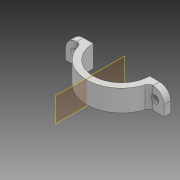
# Autodesk Inventor part: bottom_fitting
Saved by Autodesk Inventor 2017 (Build 210142000, 142)
## iProperties
Created: 2017-06-10
Part Number: bottom_fitting
Material: Generic
Document SubType Name: Modeling
Designer: ari
Density: 1 g/cm^3
Appearance: Default
Author: ari
Autodesk Inventor part; units mm, degrees
ref_plane "YZ Plane" through (0, 0, 0) normal (1, 0, 0) x (0, 1, 0)
ref_plane "XZ Plane" through (0, 0, 0) normal (0, 1, 0) x (-1, 0, 0)
ref_plane "XY Plane" through (0, 0, 0) normal (0, 0, 1) x (1, 0, 0)
sketch "Sketch1" plane through (0, 0, 0) normal (0, 0, 1) x (1, 0, 0)
  line L0 (12.7, 0) -> (22.2, 0)
  line L1 (22.2, 0) -> (22.2, -3)
  line L2 (22.2, -3) -> (12.7, -3)
  line L3 (12.7, -3) -> (12.7, 0)
  circle A0 centre (0, 0) radius 12.7
  circle A1 centre (0, 0) radius 15.7
  line L4 (-15.7, 0) -> (-12.7, 0)
  line L5 (12.7, 0) -> (15.7, 0)
  line L6 (-12.7, 0) -> (-22.2, 0)
  line L7 (-22.2, 0) -> (-22.2, -3)
  line L8 (-22.2, -3) -> (-12.7, -3)
  line L9 (-12.7, -3) -> (-12.7, 0)
  dimension "d0" = 12.7
  dimension "d1" = 3
  dimension "d2" = 3
  dimension "d3" = 6.5
  constraints: 20 end point, 4 parallel, 4 point on circle, 3 collinear, 3 horizontal, 2 centre point, 2 coincident, 2 perpendicular, 2 point on line
  measures "d0" distance from line of L3 A1.centre
  measures "d1" distance of L0.end L1.end
  measures "d2" radial gap between concentric circles of A1 A0
  measures "d3" distance edge to line of A1 L1
extrude "Extrusion1" add sketch "Sketch1" along normal blind 9.7 contours L0 A1 L2 L3 | L3 L2 A1 L8 L9 A0 | L0 L1 L2 A1 | L9 L8 A1 L4 | A1 L8 L7 L6
sketch "Sketch2" plane through (15.4107, -3, 0) normal (0, -1, 0) x (1, 0, 0)
  line L0 (0, 9.7) -> (0, 0) projected
  line L1 (0, 4.85) -> (2.75, 4.85)
  circle A0 centre (2.75, 4.85) radius 2.75
  point P0 (-15.4107, 0)
  dimension "d6" = 5.5
  constraints: 2 end point, 1 coincident, 1 horizontal, 1 horizontal alignment, 1 midpoint, 2 other
hole "Hole1" at (18.1607, -3, 4.85) direction (0, 1, 0) diameter 3.4 end through all
ref_plane "Work Plane1" through (0, -3, 0) normal (1, 0, 0) x (0, 0, -1)
mirror "Mirror1" about plane through (0, -3, 0) normal (1, 0, 0) of "Hole1"
fillet "Fillet1" radius 5 2 edges at (-22.2, -1.5, 9.7) (22.2, -1.5, 9.7)
fillet "Fillet1" radius 2 2 edges at (15.4107, -3, 4.85) (-15.4107, -3, 4.85)
body "Solid1"
